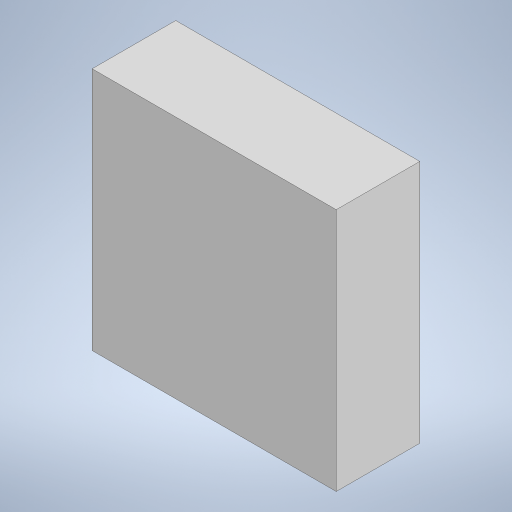
# Autodesk Inventor part: endeffectorconnector
Saved by Autodesk Inventor 2023.2 (Build 272271000, 271)
## iProperties
Created: 2022-12-19
Part Number: endeffectorconnector
Material: Generic
Document SubType Name: Modeling
Designer: omrfrkmll
Density: 1 g/cm^3
Appearance: Default
Author: omrfrkmll
Autodesk Inventor part; units mm, degrees
ref_plane "YZ Plane" through (0, 0, 0) normal (1, 0, 0) x (0, 1, 0)
ref_plane "XZ Plane" through (0, 0, 0) normal (0, 1, 0) x (-1, 0, 0)
ref_plane "XY Plane" through (0, 0, 0) normal (0, 0, 1) x (1, 0, 0)
sketch "Sketch1" plane through (0, 0, 0) normal (0, 0, 1) x (1, 0, 0)
  line L0 (0, 5.7632) -> (0, -6.6468)
  line L1 (-5.0332, 0) -> (7.4153, 0)
  line L2 (-7.3, 7.3) -> (7.3, 7.3)
  line L3 (7.3, 7.3) -> (7.3, -7.3)
  line L4 (7.3, -7.3) -> (-7.3, -7.3)
  line L5 (-7.3, -7.3) -> (-7.3, 7.3)
  point P0 (0, 0)
  dimension "d1" = 14.6
  dimension "d2" = 14.6
  constraints: 12 end point, 2 horizontal, 2 parallel, 2 point on line, 1 perpendicular, 1 vertical, 2 other
  measures "d1" distance between parallel lines of L3 L5
  measures "d2" distance between parallel lines of L4 L2
extrude "Extrusion1" add sketch "Sketch1" along normal blind 5
body "Solid1"
